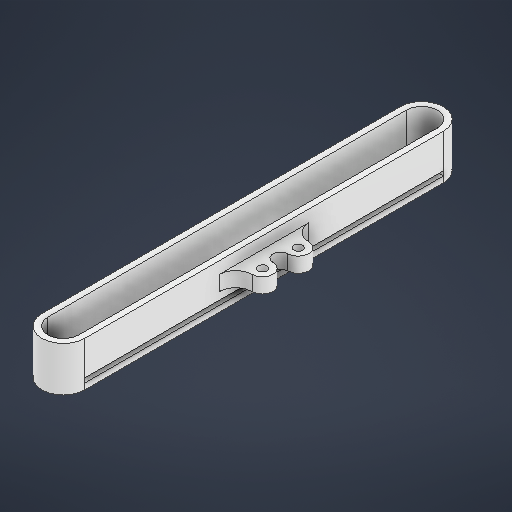
# Autodesk Inventor part: wiper_linkage_magnet_holder
Saved by Autodesk Inventor 2026.2 (Build 302298000, 298)
## iProperties
Created: 2026-03-09
Part Number: wiper_linkage_magnet_holder
Material: ABS Plastic
Document SubType Name: Modeling
Designer: Tathagata Sikdar
Density: 1.06 g/cm^3
Appearance: Smooth - White
Author: Tathagata Sikdar
Autodesk Inventor part; units mm, degrees
ref_plane "YZ Plane" through (0, 0, 0) normal (1, 0, 0) x (0, 1, 0)
ref_plane "XZ Plane" through (0, 0, 0) normal (0, 1, 0) x (-1, 0, 0)
ref_plane "XY Plane" through (0, 0, 0) normal (0, 0, 1) x (1, 0, 0)
sketch "Sketch1" plane through (0, 0, 0) normal (0, 1, 0) x (-1, 0, 0)
  line L0 (0, 0) -> (0, -130.5) construction
  line L1 (-5, -5) -> (-5, -125.5) construction
  line L2 (5, -125.5) -> (5, -5) construction
  arc A0 (5, -5) -> (-5, -5) centre (0, -5) ccw construction
  arc A1 (-5, -125.5) -> (5, -125.5) centre (0, -125.5) ccw construction
  line L3 (0, -65.25) -> (0, -71.25) construction
  line L4 (-5.2, -125.5) -> (-5.2, -5)
  arc A2 (5.2, -5) -> (-5.2, -5) centre (0, -5) ccw
  line L5 (5.2, -5) -> (5.2, -125.5)
  arc A3 (-5.2, -125.5) -> (5.2, -125.5) centre (0, -125.5) ccw
  line L6 (7.2, -125.5) -> (7.2, -5)
  arc A4 (7.2, -5) -> (-7.2, -5) centre (0, -5) ccw
  line L7 (-7.2, -5) -> (-7.2, -125.5)
  arc A5 (-7.2, -125.5) -> (7.2, -125.5) centre (0, -125.5) ccw
  line L8 (0, -71.25) -> (-12.7, -71.25) construction
  circle A6 centre (-12.7, -71.25) radius 1.5
  line L9 (-7.2, -74.75) -> (-12.7, -74.75)
  arc A7 (-12.7, -67.75) -> (-12.7, -74.75) centre (-12.7, -71.25) ccw
  line L10 (-12.7, -67.75) -> (-7.2, -67.75)
  line L11 (0, -65.25) -> (0, -59.25) construction
  line L12 (0, -59.25) -> (-7.2, -59.25) construction
  line L13 (-7.2, -59.25) -> (-12.7, -59.25) construction
  circle A8 centre (-12.7, -59.25) radius 1.5
  arc A9 (-12.7, -55.75) -> (-12.7, -62.75) centre (-12.7, -59.25) ccw
  line L14 (-12.7, -62.75) -> (-7.2, -62.75)
  line L15 (-12.7, -55.75) -> (-7.2, -55.75)
  arc A10 (-12.7, -67.75) -> (-12.7, -62.75) centre (-12.7, -65.25) ccw
  arc A11 (-7.2, -80.25) -> (-12.7, -74.75) centre (-12.7, -80.25) ccw
  arc A12 (-12.7, -55.75) -> (-7.2, -50.25) centre (-12.7, -50.25) ccw
  point P0 (-11.2, -71.25)
  point P1 (-11.2, -59.25)
  point P2 (-11.2, -59.25)
  dimension "d15" = 3
  dimension "d20" = 3
  dimension "d0" = 130.5
  dimension "d1" = 10
  dimension "d2" = 6
  dimension "d6" = 0.2
  dimension "d7" = 2
  dimension "d14" = 2
  dimension "d16" = 4
  dimension "d17" = 6
  dimension "d18" = 2
  dimension "d19" = 4
  dimension "d24" = 2.5
  constraints: 32 end point, 26 point on circle, 12 tangent, 11 centre point, 7 point on line, 6 horizontal, 4 coincident, 3 horizontal alignment, 2 parallel, 2 vertical, 2 vertical alignment, 1 midpoint, 23 other
  measures "d0" distance of L0.start L0.end
  measures "d1" diameter of A1
  measures "d2" distance of L3.start L3.end
  measures "d6" distance between parallel lines of L1 L4
  measures "d7" radial gap between concentric circles of A3 A5
  measures "d17" distance of L3.start L11.end
  measures "d24" radius of A10
extrude "Extrusion1" add sketch "Sketch1" along normal blind 1 contours L4 A2 L5 A3
extrude "Extrusion2" add sketch "Sketch1" along normal blind 15 contours A5 L7 A4 L6
ref_plane "Work Plane1" through (0, 6, 0) normal (0, -1, 0) x (1, 0, 0)
extrude "Extrusion4" add sketch "Sketch1" along normal blind 5 from surface at 6 contours A11 L9 L7 | L7 L15 A12 | L9 A7 L10 L7 | L7 L14 A9 L15 | L10 A10 L14 L7
sketch "Sketch2" plane through (7.2, 0, -5) normal (1, 0, 0) x (0, 0, -1)
  line L0 (0, 0) -> (0, 15) projected
  line L1 (120.5, 0) -> (120.5, 15) projected
  line L2 (0, 3.5) -> (120.5, 3.5)
  line L3 (120.5, 3.5) -> (120.5, 2)
  line L4 (120.5, 2) -> (0, 2)
  line L5 (0, 2) -> (0, 3.5)
  line L6 (0, 0) -> (120.5, 0) projected
  point P0 (-5, 0)
  point P1 (0, 2)
  dimension "d28" = 2
  dimension "d31" = 1.5
  constraints: 8 end point, 2 parallel, 2 point on line, 1 horizontal, 1 perpendicular
  measures "d28" distance between parallel lines of L6 L4
  measures "d31" distance between parallel lines of L4 L2
extrude "Extrusion5" cut sketch "Sketch2" against normal through all contours L0 L2 L1 L4
body "Solid1"
